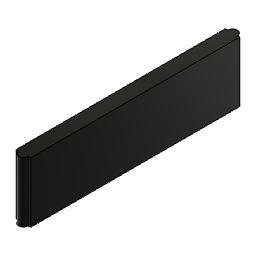
Wand (Autodesk Fusion 360 design; units mm, degrees)
Autodesk Fusion 360 part; units mm, degrees
sketch "Skizze1" plane through (0, 0, 0) normal (0, 1, 0) x (1, 0, 0)
  line L0 (0, 0) -> (6, 0)
  line L1 (6, 0) -> (6, 87)
  line L2 (6, 87) -> (0, 87)
  line L3 (0, 87) -> (0, 0)
  arc A0 (1, 0) -> (5, 0) centre (3, 0) ccw
  arc A1 (5, 87) -> (1, 87) centre (3, 87) ccw
  dimension "d1" = 87
  dimension "d2" = 6
  constraint horizontal L0
  constraint vertical L1
  constraint horizontal L2
  constraint vertical L3
  constraint coincident L0.start L3.end
  constraint coincident L0 A0.end
  constraint coincident L0 A0.start
  constraint coincident L2 A1.start
  constraint coincident L2 A1.end
  measures "d1" distance of L0.start L2.end
  measures "d2" distance of L0.start L0.end
extrude "Extrusion1" add sketch "Skizze1" along normal blind 25 makes body 1
copy_body "Körper->Berechn1" bodies 1 removing the originals makes body 2 in component "Component"
component "Component" placed x (1, 0, 0) y (0, 1, 0) z (0, 0, 1) at (0, 0, 0)
